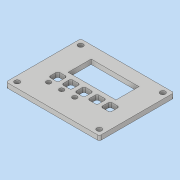
# Autodesk Inventor part: Schiled
Saved by Autodesk Inventor 2018 (Build 220112000, 112)
## iProperties
Created: 2020-10-03
Part Number: Schiled
Material: Generisch
Document SubType Name: Modeling
Designer: marce
Density: 1 g/cm^3
Appearance: Vorgabe
Author: marce
Autodesk Inventor part; units mm, degrees
ref_plane "YZ Plane" through (0, 0, 0) normal (1, 0, 0) x (0, 1, 0)
ref_plane "XZ Plane" through (0, 0, 0) normal (0, 1, 0) x (-1, 0, 0)
ref_plane "XY Plane" through (0, 0, 0) normal (0, 0, 1) x (1, 0, 0)
sketch "Skizze1" plane through (0, 0, 0) normal (0, 0, 1) x (1, 0, 0)
  line L0 (0, 0) -> (100, 0)
  line L1 (100, 0) -> (100, 80)
  line L2 (100, 80) -> (0, 80)
  line L3 (0, 80) -> (0, 0)
  dimension "d0" = 100
  dimension "d1" = 80
  constraints: 8 end point, 2 parallel, 1 horizontal, 1 perpendicular
  measures "d0" distance of L2.end L1.end
  measures "d1" distance of L1.end L0.end
extrude "Extrusion1" add sketch "Skizze1" along normal blind 5
sketch "Skizze3" plane through (0, 0, 5) normal (0, 0, 1) x (1, 0, 0)
  line L0 (15, 71) -> (85, 71)
  line L1 (85, 71) -> (85, 9)
  line L2 (85, 9) -> (15, 9)
  line L3 (15, 9) -> (15, 71)
  line L4 (100, 80) -> (0, 80) projected
  line L5 (100, 0) -> (100, 80) projected
  line L6 (24.35, 66.85) -> (75.65, 66.85)
  line L7 (75.65, 66.85) -> (75.65, 42.15)
  line L8 (75.65, 42.15) -> (24.35, 42.15)
  line L9 (24.35, 42.15) -> (24.35, 66.85)
  line L10 (18, 37.5) -> (28, 37.5)
  line L11 (28, 37.5) -> (28, 27.5)
  line L12 (28, 27.5) -> (18, 27.5)
  line L13 (18, 27.5) -> (18, 37.5)
  line L14 (23, 37.5) -> (23, 27.5)
  line L15 (18, 32.5) -> (28, 32.5)
  line L16 (32, 37.5) -> (42, 37.5)
  line L17 (42, 37.5) -> (42, 27.5)
  line L18 (42, 27.5) -> (32, 27.5)
  line L19 (32, 27.5) -> (32, 37.5)
  line L20 (46, 37.5) -> (56, 37.5)
  line L21 (56, 37.5) -> (56, 27.5)
  line L22 (56, 27.5) -> (46, 27.5)
  line L23 (46, 27.5) -> (46, 37.5)
  line L24 (60, 37.5) -> (70, 37.5)
  line L25 (70, 37.5) -> (70, 27.5)
  line L26 (70, 27.5) -> (60, 27.5)
  line L27 (60, 27.5) -> (60, 37.5)
  line L28 (74, 37.5) -> (84, 37.5)
  line L29 (84, 37.5) -> (84, 27.5)
  line L30 (84, 27.5) -> (74, 27.5)
  line L31 (74, 27.5) -> (74, 37.5)
  point P0 (0, 0)
  point P1 (85, 40)
  point P2 (100, 40)
  point P3 (50, 71)
  point P4 (50, 80)
  point P5 (50, 66.85)
  dimension "d9" = 70
  dimension "d10" = 62
  dimension "d12" = 51.3
  dimension "d13" = 24.7
  dimension "d14" = 4.15
  dimension "d15" = 10
  dimension "d16" = 10
  dimension "d21" = 8
  dimension "d22" = 23.5
  dimension "d23" = 14
  dimension "d24" = 14
  dimension "d25" = 14
  dimension "d26" = 14
  constraints: 60 end point, 14 parallel, 9 midpoint, 7 equal length, 7 horizontal, 7 perpendicular, 3 point on line, 2 collinear, 2 vertical alignment, 1 horizontal alignment
  measures "d9" distance of L1.end L2.end
  measures "d10" distance of L0.end L1.end
  measures "d12" distance of L7.end L8.end
  measures "d13" distance of L6.end L7.end
  measures "d14" distance between parallel lines of L0 L6
  measures "d15" distance of L11.end L12.end
  measures "d16" distance of L10.end L11.end
  measures "d21" distance between parallel lines of L14 L3
  measures "d22" distance between parallel lines of L2 L15
  measures "d23" distance between parallel lines of L19 L13
  measures "d24" distance between parallel lines of L23 L19
  measures "d25" distance between parallel lines of L23 L27
  measures "d26" distance between parallel lines of L27 L31
extrude "Extrusion3" cut sketch "Skizze3" against normal through all contours L6 L7 L8 L9 | L10 L14 L15 L13 | L10 L11 L15 L14 | L15 L14 L12 L13 | L15 L11 L12 L14 | L16 L17 L18 L19 | L20 L21 L22 L23 | L24 L25 L26 L27 | L28 L29 L30 L31
sketch "Skizze5" plane through (0, 0, 0) normal (0, 0, -1) x (-1, 0, 0)
  line L0 (-28, 27.5) -> (-28, 37.5) projected
  line L1 (-28, 37.5) -> (-18, 37.5) projected
  line L2 (-18, 37.5) -> (-18, 27.5) projected
  line L3 (-18, 27.5) -> (-28, 27.5) projected
  line L4 (-74, 37.5) -> (-74, 27.5) projected
  line L5 (-74, 27.5) -> (-84, 27.5) projected
  line L6 (-84, 27.5) -> (-84, 37.5) projected
  line L7 (-84, 37.5) -> (-74, 37.5) projected
  line L8 (-46, 37.5) -> (-46, 27.5) projected
  line L9 (-46, 27.5) -> (-56, 27.5) projected
  line L10 (-56, 27.5) -> (-56, 37.5) projected
  line L11 (-56, 37.5) -> (-46, 37.5) projected
  line L12 (-32, 37.5) -> (-32, 27.5) projected
  line L13 (-32, 27.5) -> (-42, 27.5) projected
  line L14 (-42, 27.5) -> (-42, 37.5) projected
  line L15 (-42, 37.5) -> (-32, 37.5) projected
  line L16 (-60, 37.5) -> (-60, 27.5) projected
  line L17 (-60, 27.5) -> (-70, 27.5) projected
  line L18 (-70, 27.5) -> (-70, 37.5) projected
  line L19 (-70, 37.5) -> (-60, 37.5) projected
  line L20 (-24.35, 66.85) -> (-24.35, 42.15) projected
  line L21 (-24.35, 42.15) -> (-75.65, 42.15) projected
  line L22 (-75.65, 42.15) -> (-75.65, 66.85) projected
  line L23 (-75.65, 66.85) -> (-24.35, 66.85) projected
  line L24 (0, 0) -> (-100, 0) projected
  line L25 (0, 80) -> (0, 0) projected
  line L26 (-100, 80) -> (0, 80) projected
  line L27 (-100, 0) -> (-100, 80) projected
  line L28 (-6, 74) -> (-6, 6)
  line L29 (-6, 6) -> (-94, 6)
  line L30 (-94, 6) -> (-94, 74)
  line L31 (-94, 74) -> (-6, 74)
  line L32 (-100, 80) -> (0, 80) projected
  dimension "d39" = 6
  constraints: 8 end point, 3 other
  measures "d39" distance between parallel lines of L32 L31
hole "Bohrung2" at (6, 74, 0) at (6, 6, 0) at (94, 6, 0) at (94, 74, 0) direction (0, 0, 1) diameter 5.5 end through all
fillet "Rundung2" radius 2 4 edges at (100, 0, 2.5) (0, 0, 2.5) (0, 80, 2.5) (100, 80, 2.5)
fillet "Rundung1" radius 2 20 edges at (18, 37.5, 2.5) (18, 27.5, 2.5) (28, 27.5, 2.5) (28, 37.5, 2.5) (32, 37.5, 2.5) (32, 27.5, 2.5) (42, 27.5, 2.5) (42, 37.5, 2.5) (46, 37.5, 2.5) (56, 37.5, 2.5) (60, 37.5, 2.5) (70, 37.5, 2.5) (74, 37.5, 2.5) (84, 37.5, 2.5) (84, 27.5, 2.5) (74, 27.5, 2.5) (70, 27.5, 2.5) (60, 27.5, 2.5) (56, 27.5, 2.5) (46, 27.5, 2.5)
sketch "Skizze4" plane through (0, 0, 0) normal (0, 0, -1) x (-1, 0, 0)
  circle A0 centre (-23.15, 22.5) radius 2.45 projected
  circle A1 centre (-37.15, 22.5) radius 2.45 projected
  circle A2 centre (-51.15, 22.5) radius 2.45 projected
  point P0 (0, 0)
hole "Bohrung1" at (51.15, 22.5, 0) at (37.15, 22.5, 0) at (23.15, 22.5, 0) direction (0, 0, 1) diameter 5 end through all
